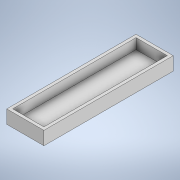
# Autodesk Inventor part: if_case_bottom
Saved by Autodesk Inventor 2020 (Build 240168000, 168)
## iProperties
Created: 2020-02-14
Part Number: if_case_bottom
Material: Generic
Document SubType Name: Modeling
Designer: mdjb501
Density: 1 g/cm^3
Appearance: Default
Author: mdjb501
Autodesk Inventor part; units mm, degrees
ref_plane "YZ Plane" through (0, 0, 0) normal (1, 0, 0) x (0, 1, 0)
ref_plane "XZ Plane" through (0, 0, 0) normal (0, 1, 0) x (-1, 0, 0)
ref_plane "XY Plane" through (0, 0, 0) normal (0, 0, 1) x (1, 0, 0)
sketch "Sketch1" plane through (0, 0, 0) normal (0, 1, 0) x (-1, 0, 0)
  line L0 (-5.25, -20.75) -> (5.25, -20.75)
  line L1 (5.25, -20.75) -> (5.25, 20.75)
  line L2 (5.25, 20.75) -> (-5.25, 20.75)
  line L3 (-5.25, 20.75) -> (-5.25, -20.75)
  line L4 (6.25, 21.75) -> (-6.25, 21.75)
  line L5 (-6.25, 21.75) -> (-6.25, -21.75)
  line L6 (-6.25, -21.75) -> (6.25, -21.75)
  line L7 (6.25, -21.75) -> (6.25, 21.75)
  point P0 (0, 0)
  constraints: 16 end point, 4 parallel, 2 horizontal, 2 perpendicular
extrude "Extrusion1" add sketch "Sketch1" along normal blind 4.5
extrude "Extrusion2" add sketch "Sketch1" along normal blind 1 contours L3 L2 L1 L0
body "Solid1"
